Autodesk Fusion 360 part; units mm, degrees
(part 3 of 5)
sketch "LED pad connection profile" plane through (0, 0, -7.475) normal (0, 0, 1) x (1, 0, 0) in component "04 Optical retainer"
  line L0 (38.5, 5.2) -> (41.5, 5.2)
  line L1 (41.5, 5.2) -> (41.5, 11.2)
  line L2 (41.5, 11.2) -> (38.5, 11.2)
  line L3 (38.5, 11.2) -> (38.5, 5.2)
  dimension "d475" = 3
  dimension "d476" = 6
  measures "d475" horizontal distance of L0.start L0.end
  measures "d476" vertical distance of L0.end L1.end
extrude "LED pad connection" add sketch "LED pad connection profile" against normal blind 1.6 separate body makes body 56 in component "04 Optical retainer"
ref_plane "WorkPlane6" through (0, 0, -7.475) normal (0, 0, 1) x (1, 0, 0) in component "04 Optical retainer"
sketch "LED pad connection profile (1)" plane through (0, 0, -7.475) normal (0, 0, 1) x (1, 0, 0) in component "04 Optical retainer"
  line L0 (38.5, 48.8) -> (41.5, 48.8)
  line L1 (41.5, 48.8) -> (41.5, 54.8)
  line L2 (41.5, 54.8) -> (38.5, 54.8)
  line L3 (38.5, 54.8) -> (38.5, 48.8)
  dimension "d481" = 3
  dimension "d482" = 6
  measures "d481" horizontal distance of L0.start L0.end
  measures "d482" vertical distance of L0.end L1.end
extrude "LED pad connection (1)" add sketch "LED pad connection profile (1)" against normal blind 1.6 separate body makes body 57 in component "04 Optical retainer"
ref_plane "WorkPlane7" through (0, 0, -4.35) normal (0, 0, 1) x (1, 0, 0) in component "04 Optical retainer"
sketch "LED hold-down pad profile" plane through (0, 0, -4.35) normal (0, 0, 1) x (1, 0, 0) in component "04 Optical retainer"
  line L0 (38.5, 5.2) -> (41.5, 5.2)
  line L1 (41.5, 5.2) -> (41.5, 10.8)
  line L2 (41.5, 10.8) -> (38.5, 10.8)
  line L3 (38.5, 10.8) -> (38.5, 5.2)
  dimension "d487" = 3
  dimension "d488" = 5.6
  measures "d487" horizontal distance of L0.start L0.end
  measures "d488" vertical distance of L0.end L1.end
extrude "LED hold-down pad" add sketch "LED hold-down pad profile" against normal blind 3.125 separate body makes body 58 in component "04 Optical retainer"
ref_plane "WorkPlane8" through (0, 0, -4.35) normal (0, 0, 1) x (1, 0, 0) in component "04 Optical retainer"
sketch "LED hold-down pad profile (1)" plane through (0, 0, -4.35) normal (0, 0, 1) x (1, 0, 0) in component "04 Optical retainer"
  line L0 (38.5, 49.2) -> (41.5, 49.2)
  line L1 (41.5, 49.2) -> (41.5, 54.8)
  line L2 (41.5, 54.8) -> (38.5, 54.8)
  line L3 (38.5, 54.8) -> (38.5, 49.2)
  dimension "d493" = 3
  dimension "d494" = 5.6
  measures "d493" horizontal distance of L0.start L0.end
  measures "d494" vertical distance of L0.end L1.end
extrude "LED hold-down pad (1)" add sketch "LED hold-down pad profile (1)" against normal blind 3.125 separate body makes body 59 in component "04 Optical retainer"
ref_plane "WorkPlane9" through (0, 0, -7.475) normal (0, 0, 1) x (1, 0, 0) in component "04 Optical retainer"
sketch "LED pad connection profile (2)" plane through (0, 0, -7.475) normal (0, 0, 1) x (1, 0, 0) in component "04 Optical retainer"
  line L0 (78.5, 5.2) -> (81.5, 5.2)
  line L1 (81.5, 5.2) -> (81.5, 11.2)
  line L2 (81.5, 11.2) -> (78.5, 11.2)
  line L3 (78.5, 11.2) -> (78.5, 5.2)
  dimension "d499" = 3
  dimension "d500" = 6
  measures "d499" horizontal distance of L0.start L0.end
  measures "d500" vertical distance of L0.end L1.end
extrude "LED pad connection (2)" add sketch "LED pad connection profile (2)" against normal blind 1.6 separate body makes body 60 in component "04 Optical retainer"
ref_plane "WorkPlane10" through (0, 0, -7.475) normal (0, 0, 1) x (1, 0, 0) in component "04 Optical retainer"
sketch "LED pad connection profile (3)" plane through (0, 0, -7.475) normal (0, 0, 1) x (1, 0, 0) in component "04 Optical retainer"
  line L0 (78.5, 48.8) -> (81.5, 48.8)
  line L1 (81.5, 48.8) -> (81.5, 54.8)
  line L2 (81.5, 54.8) -> (78.5, 54.8)
  line L3 (78.5, 54.8) -> (78.5, 48.8)
  dimension "d505" = 3
  dimension "d506" = 6
  measures "d505" horizontal distance of L0.start L0.end
  measures "d506" vertical distance of L0.end L1.end
extrude "LED pad connection (3)" add sketch "LED pad connection profile (3)" against normal blind 1.6 separate body makes body 61 in component "04 Optical retainer"
ref_plane "WorkPlane11" through (0, 0, -4.35) normal (0, 0, 1) x (1, 0, 0) in component "04 Optical retainer"
sketch "LED hold-down pad profile (2)" plane through (0, 0, -4.35) normal (0, 0, 1) x (1, 0, 0) in component "04 Optical retainer"
  line L0 (78.5, 5.2) -> (81.5, 5.2)
  line L1 (81.5, 5.2) -> (81.5, 10.8)
  line L2 (81.5, 10.8) -> (78.5, 10.8)
  line L3 (78.5, 10.8) -> (78.5, 5.2)
  dimension "d511" = 3
  dimension "d512" = 5.6
  measures "d511" horizontal distance of L0.start L0.end
  measures "d512" vertical distance of L0.end L1.end
extrude "LED hold-down pad (2)" add sketch "LED hold-down pad profile (2)" against normal blind 3.125 separate body makes body 62 in component "04 Optical retainer"
ref_plane "WorkPlane12" through (0, 0, -4.35) normal (0, 0, 1) x (1, 0, 0) in component "04 Optical retainer"
sketch "LED hold-down pad profile (3)" plane through (0, 0, -4.35) normal (0, 0, 1) x (1, 0, 0) in component "04 Optical retainer"
  line L0 (78.5, 49.2) -> (81.5, 49.2)
  line L1 (81.5, 49.2) -> (81.5, 54.8)
  line L2 (81.5, 54.8) -> (78.5, 54.8)
  line L3 (78.5, 54.8) -> (78.5, 49.2)
  dimension "d517" = 3
  dimension "d518" = 5.6
  measures "d517" horizontal distance of L0.start L0.end
  measures "d518" vertical distance of L0.end L1.end
extrude "LED hold-down pad (3)" add sketch "LED hold-down pad profile (3)" against normal blind 3.125 separate body makes body 63 in component "04 Optical retainer"
combine "Union manufactured solid''" operation add target body 53 tool bodies 54 55 56 57 58 59 60 61 62 63 in component "04 Optical retainer"
ref_plane "WorkPlane13" through (0, 0, -7.455) normal (0, 0, 1) x (1, 0, 0) in component "04 Optical retainer"
sketch "Optical M3 clearance profile" plane through (0, 0, -7.455) normal (0, 0, 1) x (1, 0, 0) in component "04 Optical retainer"
  circle A0 centre (60, 6) radius 1.7
  dimension "d523" = 3.4
  measures "d523" diameter of A0
extrude "Optical M3 clearance" cut sketch "Optical M3 clearance profile" against normal blind 1.64 bodies 53 in component "04 Optical retainer"
ref_plane "WorkPlane14" through (0, 0, -7.455) normal (0, 0, 1) x (1, 0, 0) in component "04 Optical retainer"
sketch "Optical M3 clearance profile (1)" plane through (0, 0, -7.455) normal (0, 0, 1) x (1, 0, 0) in component "04 Optical retainer"
  circle A0 centre (60, 54) radius 1.7
  dimension "d528" = 3.4
  measures "d528" diameter of A0
extrude "Optical M3 clearance (1)" cut sketch "Optical M3 clearance profile (1)" against normal blind 1.64 bodies 53 in component "04 Optical retainer"
ref_plane "WorkPlane1" through (0, 0, -4.775) normal (0, 0, 1) x (1, 0, 0) in component "81 Laminate front spacer"
sketch "Laminate front spacer" plane through (0, 0, -4.775) normal (0, 0, 1) x (1, 0, 0) in component "81 Laminate front spacer"
  line L0 (8, 11) -> (112, 11)
  line L1 (112, 11) -> (112, 49)
  line L2 (112, 49) -> (11, 49)
  line L3 (11, 49) -> (8, 46)
  line L4 (8, 46) -> (8, 11)
extrude "Laminate front spacer (1)" add sketch "Laminate front spacer" against normal blind 0.5 separate body makes body 64 in component "81 Laminate front spacer"
ref_plane "WorkPlane2" through (0, 0, -4.765) normal (0, 0, 1) x (1, 0, 0) in component "81 Laminate front spacer"
sketch "Hidden border opening profile" plane through (0, 0, -4.765) normal (0, 0, 1) x (1, 0, 0) in component "81 Laminate front spacer"
  line L0 (9.5, 12.5) -> (110.5, 12.5)
  line L1 (110.5, 12.5) -> (110.5, 47.5)
  line L2 (110.5, 47.5) -> (9.5, 47.5)
  line L3 (9.5, 47.5) -> (9.5, 12.5)
  dimension "d537" = 101
  dimension "d538" = 35
  measures "d537" horizontal distance of L0.start L0.end
  measures "d538" vertical distance of L0.end L1.end
extrude "Hidden border opening" cut sketch "Hidden border opening profile" against normal blind 0.52 bodies 64 in component "81 Laminate front spacer"
ref_plane "WorkPlane1" through (0, 0, -6.875) normal (0, 0, 1) x (1, 0, 0) in component "82 Laminate rear shim"
sketch "Laminate rear shim" plane through (0, 0, -6.875) normal (0, 0, 1) x (1, 0, 0) in component "82 Laminate rear shim"
  line L0 (8, 11) -> (112, 11)
  line L1 (112, 11) -> (112, 49)
  line L2 (112, 49) -> (11, 49)
  line L3 (11, 49) -> (8, 46)
  line L4 (8, 46) -> (8, 11)
extrude "Laminate rear shim (1)" add sketch "Laminate rear shim" against normal blind 0.4 separate body makes body 65 in component "82 Laminate rear shim"
ref_plane "WorkPlane2" through (0, 0, -6.865) normal (0, 0, 1) x (1, 0, 0) in component "82 Laminate rear shim"
sketch "Hidden border opening profile (2)" plane through (0, 0, -6.865) normal (0, 0, 1) x (1, 0, 0) in component "82 Laminate rear shim"
  line L0 (9.5, 12.5) -> (110.5, 12.5)
  line L1 (110.5, 12.5) -> (110.5, 47.5)
  line L2 (110.5, 47.5) -> (9.5, 47.5)
  line L3 (9.5, 47.5) -> (9.5, 12.5)
  dimension "d547" = 101
  dimension "d548" = 35
  measures "d547" horizontal distance of L0.start L0.end
  measures "d548" vertical distance of L0.end L1.end
extrude "Hidden border opening'" cut sketch "Hidden border opening profile (2)" against normal blind 0.42 bodies 65 in component "82 Laminate rear shim"
ref_plane "WorkPlane1" through (0, 0, -9.5) normal (0, 0, 1) x (1, 0, 0) in component "05 Rear electronics housing"
sketch "Rear housing envelope profile" plane through (0, 0, -9.5) normal (0, 0, 1) x (1, 0, 0) in component "05 Rear electronics housing"
  line L0 (3, 0) -> (117, 0)
  line L1 (120, 3) -> (120, 57)
  line L2 (117, 60) -> (3, 60)
  line L3 (0, 57) -> (0, 3)
  arc A0 (117, 0) -> (120, 3) centre (117, 3) ccw
  arc A1 (120, 57) -> (117, 60) centre (117, 57) ccw
  arc A2 (3, 60) -> (0, 57) centre (3, 57) ccw
  arc A3 (0, 3) -> (3, 0) centre (3, 3) ccw
extrude "Rear housing envelope" add sketch "Rear housing envelope profile" against normal blind 24.5 separate body makes body 66 in component "05 Rear electronics housing"
ref_plane "WorkPlane2" through (0, 0, -9.48) normal (0, 0, 1) x (1, 0, 0) in component "05 Rear electronics housing"
sketch "Front open electronics cavity profile" plane through (0, 0, -9.48) normal (0, 0, 1) x (1, 0, 0) in component "05 Rear electronics housing"
  line L0 (2.4, 2.4) -> (117.6, 2.4)
  line L1 (117.6, 2.4) -> (117.6, 57.6)
  line L2 (117.6, 57.6) -> (2.4, 57.6)
  line L3 (2.4, 57.6) -> (2.4, 2.4)
  dimension "d557" = 115.2
  dimension "d558" = 55.2
  measures "d557" horizontal distance of L0.start L0.end
  measures "d558" vertical distance of L0.end L1.end
extrude "Front open electronics cavity" cut sketch "Front open electronics cavity profile" against normal blind 22.12 bodies 66 in component "05 Rear electronics housing"
ref_plane "WorkPlane3" through (0, 0, -9.5) normal (0, 0, 1) x (1, 0, 0) in component "05 Rear electronics housing"
sketch "Closure boss profile" plane through (0, 0, -9.5) normal (0, 0, 1) x (1, 0, 0) in component "05 Rear electronics housing"
  line L0 (1.8, 1.8) -> (10.2, 1.8)
  line L1 (10.2, 1.8) -> (10.2, 10.2)
  line L2 (10.2, 10.2) -> (1.8, 10.2)
  line L3 (1.8, 10.2) -> (1.8, 1.8)
  dimension "d563" = 8.4
  dimension "d564" = 8.4
  measures "d563" horizontal distance of L0.start L0.end
  measures "d564" vertical distance of L0.end L1.end
extrude "Closure boss" add sketch "Closure boss profile" against normal blind 22.2 separate body makes body 67 in component "05 Rear electronics housing"
combine "Union manufactured solid'''" operation add target body 66 tool bodies 67 in component "05 Rear electronics housing"
ref_plane "WorkPlane4" through (0, 0, -24.8) normal (0, 0, 1) x (1, 0, 0) in component "05 Rear electronics housing"
sketch "Closure boss hex pocket" plane through (0, 0, -24.8) normal (0, 0, 1) x (1, 0, 0) in component "05 Rear electronics housing"
  line L0 (9.3486, 6) -> (7.6743, 8.9)
  line L1 (7.6743, 8.9) -> (4.3257, 8.9)
  line L2 (4.3257, 8.9) -> (2.6514, 6)
  line L3 (2.6514, 6) -> (4.3257, 3.1)
  line L4 (4.3257, 3.1) -> (7.6743, 3.1)
  line L5 (7.6743, 3.1) -> (9.3486, 6)
extrude "Closure boss hex pocket (1)" cut sketch "Closure boss hex pocket" against normal blind 2.6 bodies 66 in component "05 Rear electronics housing"
ref_plane "WorkPlane5" through (0, 0, -24.8) normal (0, 0, 1) x (1, 0, 0) in component "05 Rear electronics housing"
sketch "Closure boss side nut entry profile" plane through (0, 0, -24.8) normal (0, 0, 1) x (1, 0, 0) in component "05 Rear electronics housing"
  line L0 (6, 3.1) -> (10.5, 3.1)
  line L1 (10.5, 3.1) -> (10.5, 8.9)
  line L2 (10.5, 8.9) -> (6, 8.9)
  line L3 (6, 8.9) -> (6, 3.1)
  dimension "d573" = 4.5
  dimension "d574" = 5.8
  measures "d573" horizontal distance of L0.start L0.end
  measures "d574" vertical distance of L0.end L1.end
extrude "Closure boss side nut entry" cut sketch "Closure boss side nut entry profile" against normal blind 2.6 bodies 66 in component "05 Rear electronics housing"
ref_plane "WorkPlane6" through (0, 0, -9.48) normal (0, 0, 1) x (1, 0, 0) in component "05 Rear electronics housing"
sketch "Closure boss blind bore profile" plane through (0, 0, -9.48) normal (0, 0, 1) x (1, 0, 0) in component "05 Rear electronics housing"
  circle A0 centre (6, 6) radius 1.7
  dimension "d579" = 3.4
  measures "d579" diameter of A0
extrude "Closure boss blind bore" cut sketch "Closure boss blind bore profile" against normal blind 19.72 bodies 66 in component "05 Rear electronics housing"
ref_plane "WorkPlane7" through (0, 0, -9.5) normal (0, 0, 1) x (1, 0, 0) in component "05 Rear electronics housing"
sketch "Closure boss profile (1)" plane through (0, 0, -9.5) normal (0, 0, 1) x (1, 0, 0) in component "05 Rear electronics housing"
  line L0 (109.8, 1.8) -> (118.2, 1.8)
  line L1 (118.2, 1.8) -> (118.2, 10.2)
  line L2 (118.2, 10.2) -> (109.8, 10.2)
  line L3 (109.8, 10.2) -> (109.8, 1.8)
  dimension "d584" = 8.4
  dimension "d585" = 8.4
  measures "d584" horizontal distance of L0.start L0.end
  measures "d585" vertical distance of L0.end L1.end
extrude "Closure boss (1)" add sketch "Closure boss profile (1)" against normal blind 22.2 separate body makes body 68 in component "05 Rear electronics housing"
combine "Union manufactured solid (1)''" operation add target body 66 tool bodies 68 in component "05 Rear electronics housing"
ref_plane "WorkPlane8" through (0, 0, -24.8) normal (0, 0, 1) x (1, 0, 0) in component "05 Rear electronics housing"
sketch "Closure boss hex pocket (1)" plane through (0, 0, -24.8) normal (0, 0, 1) x (1, 0, 0) in component "05 Rear electronics housing"
  line L0 (117.3486, 6) -> (115.6743, 8.9)
  line L1 (115.6743, 8.9) -> (112.3257, 8.9)
  line L2 (112.3257, 8.9) -> (110.6514, 6)
  line L3 (110.6514, 6) -> (112.3257, 3.1)
  line L4 (112.3257, 3.1) -> (115.6743, 3.1)
  line L5 (115.6743, 3.1) -> (117.3486, 6)
extrude "Closure boss hex pocket (2)" cut sketch "Closure boss hex pocket (1)" against normal blind 2.6 bodies 66 in component "05 Rear electronics housing"
ref_plane "WorkPlane9" through (0, 0, -24.8) normal (0, 0, 1) x (1, 0, 0) in component "05 Rear electronics housing"
sketch "Closure boss side nut entry profile (1)" plane through (0, 0, -24.8) normal (0, 0, 1) x (1, 0, 0) in component "05 Rear electronics housing"
  line L0 (109.5, 3.1) -> (114, 3.1)
  line L1 (114, 3.1) -> (114, 8.9)
  line L2 (114, 8.9) -> (109.5, 8.9)
  line L3 (109.5, 8.9) -> (109.5, 3.1)
  dimension "d594" = 4.5
  dimension "d595" = 5.8
  measures "d594" horizontal distance of L0.start L0.end
  measures "d595" vertical distance of L0.end L1.end
extrude "Closure boss side nut entry (1)" cut sketch "Closure boss side nut entry profile (1)" against normal blind 2.6 bodies 66 in component "05 Rear electronics housing"
ref_plane "WorkPlane10" through (0, 0, -9.48) normal (0, 0, 1) x (1, 0, 0) in component "05 Rear electronics housing"
sketch "Closure boss blind bore profile (1)" plane through (0, 0, -9.48) normal (0, 0, 1) x (1, 0, 0) in component "05 Rear electronics housing"
  circle A0 centre (114, 6) radius 1.7
  dimension "d600" = 3.4
  measures "d600" diameter of A0
extrude "Closure boss blind bore (1)" cut sketch "Closure boss blind bore profile (1)" against normal blind 19.72 bodies 66 in component "05 Rear electronics housing"
ref_plane "WorkPlane11" through (0, 0, -9.5) normal (0, 0, 1) x (1, 0, 0) in component "05 Rear electronics housing"
sketch "Closure boss profile (2)" plane through (0, 0, -9.5) normal (0, 0, 1) x (1, 0, 0) in component "05 Rear electronics housing"
  line L0 (1.8, 49.8) -> (10.2, 49.8)
  line L1 (10.2, 49.8) -> (10.2, 58.2)
  line L2 (10.2, 58.2) -> (1.8, 58.2)
  line L3 (1.8, 58.2) -> (1.8, 49.8)
  dimension "d605" = 8.4
  dimension "d606" = 8.4
  measures "d605" horizontal distance of L0.start L0.end
  measures "d606" vertical distance of L0.end L1.end
extrude "Closure boss (2)" add sketch "Closure boss profile (2)" against normal blind 22.2 separate body makes body 69 in component "05 Rear electronics housing"
combine "Union manufactured solid (2)'" operation add target body 66 tool bodies 69 in component "05 Rear electronics housing"
ref_plane "WorkPlane12" through (0, 0, -24.8) normal (0, 0, 1) x (1, 0, 0) in component "05 Rear electronics housing"
sketch "Closure boss hex pocket (2)" plane through (0, 0, -24.8) normal (0, 0, 1) x (1, 0, 0) in component "05 Rear electronics housing"
  line L0 (9.3486, 54) -> (7.6743, 56.9)
  line L1 (7.6743, 56.9) -> (4.3257, 56.9)
  line L2 (4.3257, 56.9) -> (2.6514, 54)
  line L3 (2.6514, 54) -> (4.3257, 51.1)
  line L4 (4.3257, 51.1) -> (7.6743, 51.1)
  line L5 (7.6743, 51.1) -> (9.3486, 54)
extrude "Closure boss hex pocket (3)" cut sketch "Closure boss hex pocket (2)" against normal blind 2.6 bodies 66 in component "05 Rear electronics housing"
ref_plane "WorkPlane13" through (0, 0, -24.8) normal (0, 0, 1) x (1, 0, 0) in component "05 Rear electronics housing"
sketch "Closure boss side nut entry profile (2)" plane through (0, 0, -24.8) normal (0, 0, 1) x (1, 0, 0) in component "05 Rear electronics housing"
  line L0 (6, 51.1) -> (10.5, 51.1)
  line L1 (10.5, 51.1) -> (10.5, 56.9)
  line L2 (10.5, 56.9) -> (6, 56.9)
  line L3 (6, 56.9) -> (6, 51.1)
  dimension "d615" = 4.5
  dimension "d616" = 5.8
  measures "d615" horizontal distance of L0.start L0.end
  measures "d616" vertical distance of L0.end L1.end
extrude "Closure boss side nut entry (2)" cut sketch "Closure boss side nut entry profile (2)" against normal blind 2.6 bodies 66 in component "05 Rear electronics housing"
ref_plane "WorkPlane14" through (0, 0, -9.48) normal (0, 0, 1) x (1, 0, 0) in component "05 Rear electronics housing"
sketch "Closure boss blind bore profile (2)" plane through (0, 0, -9.48) normal (0, 0, 1) x (1, 0, 0) in component "05 Rear electronics housing"
  circle A0 centre (6, 54) radius 1.7
  dimension "d621" = 3.4
  measures "d621" diameter of A0
extrude "Closure boss blind bore (2)" cut sketch "Closure boss blind bore profile (2)" against normal blind 19.72 bodies 66 in component "05 Rear electronics housing"
ref_plane "WorkPlane15" through (0, 0, -9.5) normal (0, 0, 1) x (1, 0, 0) in component "05 Rear electronics housing"
sketch "Closure boss profile (3)" plane through (0, 0, -9.5) normal (0, 0, 1) x (1, 0, 0) in component "05 Rear electronics housing"
  line L0 (91.8, 49.8) -> (100.2, 49.8)
  line L1 (100.2, 49.8) -> (100.2, 58.2)
  line L2 (100.2, 58.2) -> (91.8, 58.2)
  line L3 (91.8, 58.2) -> (91.8, 49.8)
  dimension "d626" = 8.4
  dimension "d627" = 8.4
  measures "d626" horizontal distance of L0.start L0.end
  measures "d627" vertical distance of L0.end L1.end
extrude "Closure boss (3)" add sketch "Closure boss profile (3)" against normal blind 22.2 separate body makes body 70 in component "05 Rear electronics housing"
combine "Union manufactured solid (3)" operation add target body 66 tool bodies 70 in component "05 Rear electronics housing"
ref_plane "WorkPlane16" through (0, 0, -24.8) normal (0, 0, 1) x (1, 0, 0) in component "05 Rear electronics housing"
sketch "Closure boss hex pocket (3)" plane through (0, 0, -24.8) normal (0, 0, 1) x (1, 0, 0) in component "05 Rear electronics housing"
  line L0 (99.3486, 54) -> (97.6743, 56.9)
  line L1 (97.6743, 56.9) -> (94.3257, 56.9)
  line L2 (94.3257, 56.9) -> (92.6514, 54)
  line L3 (92.6514, 54) -> (94.3257, 51.1)
  line L4 (94.3257, 51.1) -> (97.6743, 51.1)
  line L5 (97.6743, 51.1) -> (99.3486, 54)
extrude "Closure boss hex pocket (4)" cut sketch "Closure boss hex pocket (3)" against normal blind 2.6 bodies 66 in component "05 Rear electronics housing"
ref_plane "WorkPlane17" through (0, 0, -24.8) normal (0, 0, 1) x (1, 0, 0) in component "05 Rear electronics housing"
sketch "Closure boss side nut entry profile (3)" plane through (0, 0, -24.8) normal (0, 0, 1) x (1, 0, 0) in component "05 Rear electronics housing"
  line L0 (91.5, 51.1) -> (96, 51.1)
  line L1 (96, 51.1) -> (96, 56.9)
  line L2 (96, 56.9) -> (91.5, 56.9)
  line L3 (91.5, 56.9) -> (91.5, 51.1)
  dimension "d636" = 4.5
  dimension "d637" = 5.8
  measures "d636" horizontal distance of L0.start L0.end
  measures "d637" vertical distance of L0.end L1.end
extrude "Closure boss side nut entry (3)" cut sketch "Closure boss side nut entry profile (3)" against normal blind 2.6 bodies 66 in component "05 Rear electronics housing"
ref_plane "WorkPlane18" through (0, 0, -9.48) normal (0, 0, 1) x (1, 0, 0) in component "05 Rear electronics housing"
sketch "Closure boss blind bore profile (3)" plane through (0, 0, -9.48) normal (0, 0, 1) x (1, 0, 0) in component "05 Rear electronics housing"
  circle A0 centre (96, 54) radius 1.7
  dimension "d642" = 3.4
  measures "d642" diameter of A0
extrude "Closure boss blind bore (3)" cut sketch "Closure boss blind bore profile (3)" against normal blind 19.72 bodies 66 in component "05 Rear electronics housing"
ref_plane "WorkPlane19" through (0, 0, -27.1) normal (0, 0, 1) x (1, 0, 0) in component "05 Rear electronics housing"
sketch "Battery fence profile" plane through (0, 0, -27.1) normal (0, 0, 1) x (1, 0, 0) in component "05 Rear electronics housing"
  line L0 (32.4, 8.4) -> (89.6, 8.4)
  line L1 (89.6, 8.4) -> (89.6, 10)
  line L2 (89.6, 10) -> (32.4, 10)
  line L3 (32.4, 10) -> (32.4, 8.4)
  dimension "d647" = 57.2
  dimension "d648" = 1.6
  measures "d647" horizontal distance of L0.start L0.end
  measures "d648" vertical distance of L0.end L1.end
extrude "Battery fence" add sketch "Battery fence profile" against normal blind 4.6 separate body makes body 71 in component "05 Rear electronics housing"
ref_plane "WorkPlane20" through (0, 0, -27.1) normal (0, 0, 1) x (1, 0, 0) in component "05 Rear electronics housing"
sketch "Battery fence profile (1)" plane through (0, 0, -27.1) normal (0, 0, 1) x (1, 0, 0) in component "05 Rear electronics housing"
  line L0 (32.4, 10) -> (34, 10)
  line L1 (34, 10) -> (34, 33)
  line L2 (34, 33) -> (32.4, 33)
  line L3 (32.4, 33) -> (32.4, 10)
  dimension "d653" = 1.6
  dimension "d654" = 23
  measures "d653" horizontal distance of L0.start L0.end
  measures "d654" vertical distance of L0.end L1.end
extrude "Battery fence (1)" add sketch "Battery fence profile (1)" against normal blind 4.6 separate body makes body 72 in component "05 Rear electronics housing"
ref_plane "WorkPlane21" through (0, 0, -27.1) normal (0, 0, 1) x (1, 0, 0) in component "05 Rear electronics housing"
sketch "Battery fence profile (2)" plane through (0, 0, -27.1) normal (0, 0, 1) x (1, 0, 0) in component "05 Rear electronics housing"
  line L0 (88, 10) -> (89.6, 10)
  line L1 (89.6, 10) -> (89.6, 27)
  line L2 (89.6, 27) -> (88, 27)
  line L3 (88, 27) -> (88, 10)
  dimension "d659" = 1.6
  dimension "d660" = 17
  measures "d659" horizontal distance of L0.start L0.end
  measures "d660" vertical distance of L0.end L1.end
extrude "Battery fence (2)" add sketch "Battery fence profile (2)" against normal blind 4.6 separate body makes body 73 in component "05 Rear electronics housing"
ref_plane "WorkPlane22" through (0, 0, -27.1) normal (0, 0, 1) x (1, 0, 0) in component "05 Rear electronics housing"
sketch "Battery fence profile (3)" plane through (0, 0, -27.1) normal (0, 0, 1) x (1, 0, 0) in component "05 Rear electronics housing"
  line L0 (34, 33) -> (74, 33)
  line L1 (74, 33) -> (74, 34.6)
  line L2 (74, 34.6) -> (34, 34.6)
  line L3 (34, 34.6) -> (34, 33)
  dimension "d665" = 40
  dimension "d666" = 1.6
  measures "d665" horizontal distance of L0.start L0.end
  measures "d666" vertical distance of L0.end L1.end
extrude "Battery fence (3)" add sketch "Battery fence profile (3)" against normal blind 4.6 separate body makes body 74 in component "05 Rear electronics housing"
ref_plane "WorkPlane23" through (0, 0, -31.3) normal (0, 0, 1) x (1, 0, 0) in component "05 Rear electronics housing"
sketch "Battery bed profile" plane through (0, 0, -31.3) normal (0, 0, 1) x (1, 0, 0) in component "05 Rear electronics housing"
  line L0 (34, 10) -> (88, 10)
  line L1 (88, 10) -> (88, 33)
  line L2 (88, 33) -> (34, 33)
  line L3 (34, 33) -> (34, 10)
  dimension "d671" = 54
  dimension "d672" = 23
  measures "d671" horizontal distance of L0.start L0.end
  measures "d672" vertical distance of L0.end L1.end
extrude "Battery bed" add sketch "Battery bed profile" against normal blind 0.4 separate body makes body 75 in component "05 Rear electronics housing"
ref_plane "WorkPlane24" through (0, 0, -25.2) normal (0, 0, 1) x (1, 0, 0) in component "05 Rear electronics housing"
sketch "Raised strap lug profile" plane through (0, 0, -25.2) normal (0, 0, 1) x (1, 0, 0) in component "05 Rear electronics housing"
  line L0 (28.4, 18) -> (32.4, 18)
  line L1 (32.4, 18) -> (32.4, 25)
  line L2 (32.4, 25) -> (28.4, 25)
  line L3 (28.4, 25) -> (28.4, 18)
  dimension "d677" = 4
  dimension "d678" = 7
  measures "d677" horizontal distance of L0.start L0.end
  measures "d678" vertical distance of L0.end L1.end
extrude "Raised strap lug" add sketch "Raised strap lug profile" against normal blind 6.5 separate body makes body 76 in component "05 Rear electronics housing"
ref_plane "WorkPlane25" through (0, 0, -25.2) normal (0, 0, 1) x (1, 0, 0) in component "05 Rear electronics housing"
sketch "Raised strap lug profile (1)" plane through (0, 0, -25.2) normal (0, 0, 1) x (1, 0, 0) in component "05 Rear electronics housing"
  line L0 (90, 18) -> (94, 18)
  line L1 (94, 18) -> (94, 25)
  line L2 (94, 25) -> (90, 25)
  line L3 (90, 25) -> (90, 18)
  dimension "d683" = 4
  dimension "d684" = 7
  measures "d683" horizontal distance of L0.start L0.end
  measures "d684" vertical distance of L0.end L1.end
extrude "Raised strap lug (1)" add sketch "Raised strap lug profile (1)" against normal blind 6.5 separate body makes body 77 in component "05 Rear electronics housing"
combine "Union manufactured solid (4)" operation add target body 66 tool bodies 71 72 73 74 75 76 77 in component "05 Rear electronics housing"
ref_plane "WorkPlane26" through (28.3, 0, 0) normal (1, 0, 0) x (0, 1, 0) in component "05 Rear electronics housing"
sketch "Strap slot with tent roof" plane through (28.3, 0, 0) normal (1, 0, 0) x (0, 0, -1) in component "05 Rear electronics housing"
  line L0 (30.4, 20) -> (30.4, 23)
  line L1 (30.4, 23) -> (28.8, 23)
  line L2 (28.8, 23) -> (27.3, 21.5)
  line L3 (27.3, 21.5) -> (28.8, 20)
  line L4 (28.8, 20) -> (30.4, 20)
extrude "Strap slot with tent roof (1)" cut sketch "Strap slot with tent roof" along normal blind 4.2 bodies 66 in component "05 Rear electronics housing"
ref_plane "WorkPlane27" through (89.9, 0, 0) normal (1, 0, 0) x (0, 1, 0) in component "05 Rear electronics housing"
sketch "Strap slot with tent roof (1)" plane through (89.9, 0, 0) normal (1, 0, 0) x (0, 0, -1) in component "05 Rear electronics housing"
  line L0 (30.4, 20) -> (30.4, 23)
  line L1 (30.4, 23) -> (28.8, 23)
  line L2 (28.8, 23) -> (27.3, 21.5)
  line L3 (27.3, 21.5) -> (28.8, 20)
  line L4 (28.8, 20) -> (30.4, 20)
extrude "Strap slot with tent roof (2)" cut sketch "Strap slot with tent roof (1)" along normal blind 4.2 bodies 66 in component "05 Rear electronics housing"
ref_plane "WorkPlane28" through (0, 0, -24.2) normal (0, 0, 1) x (1, 0, 0) in component "05 Rear electronics housing"
sketch "Charger PCB seat profile" plane through (0, 0, -24.2) normal (0, 0, 1) x (1, 0, 0) in component "05 Rear electronics housing"
  line L0 (13.1, 34) -> (15.1, 34)
  line L1 (15.1, 34) -> (15.1, 36)
  line L2 (15.1, 36) -> (13.1, 36)
  line L3 (13.1, 36) -> (13.1, 34)
  dimension "d697" = 2
  dimension "d698" = 2
  measures "d697" horizontal distance of L0.start L0.end
  measures "d698" vertical distance of L0.end L1.end
extrude "Charger PCB seat" add sketch "Charger PCB seat profile" against normal blind 7.5 separate body makes body 78 in component "05 Rear electronics housing"
ref_plane "WorkPlane29" through (0, 0, -24.2) normal (0, 0, 1) x (1, 0, 0) in component "05 Rear electronics housing"
sketch "Charger PCB seat profile (1)" plane through (0, 0, -24.2) normal (0, 0, 1) x (1, 0, 0) in component "05 Rear electronics housing"
  line L0 (26.9, 34) -> (28.9, 34)
  line L1 (28.9, 34) -> (28.9, 36)
  line L2 (28.9, 36) -> (26.9, 36)
  line L3 (26.9, 36) -> (26.9, 34)
  dimension "d703" = 2
  dimension "d704" = 2
  measures "d703" horizontal distance of L0.start L0.end
  measures "d704" vertical distance of L0.end L1.end
extrude "Charger PCB seat (1)" add sketch "Charger PCB seat profile (1)" against normal blind 7.5 separate body makes body 79 in component "05 Rear electronics housing"
ref_plane "WorkPlane30" through (0, 0, -24.2) normal (0, 0, 1) x (1, 0, 0) in component "05 Rear electronics housing"
sketch "Charger PCB seat profile (2)" plane through (0, 0, -24.2) normal (0, 0, 1) x (1, 0, 0) in component "05 Rear electronics housing"
  line L0 (13.1, 51) -> (15.1, 51)
  line L1 (15.1, 51) -> (15.1, 53)
  line L2 (15.1, 53) -> (13.1, 53)
  line L3 (13.1, 53) -> (13.1, 51)
  dimension "d709" = 2
  dimension "d710" = 2
  measures "d709" horizontal distance of L0.start L0.end
  measures "d710" vertical distance of L0.end L1.end
extrude "Charger PCB seat (2)" add sketch "Charger PCB seat profile (2)" against normal blind 7.5 separate body makes body 80 in component "05 Rear electronics housing"
ref_plane "WorkPlane31" through (0, 0, -24.2) normal (0, 0, 1) x (1, 0, 0) in component "05 Rear electronics housing"
sketch "Charger PCB seat profile (3)" plane through (0, 0, -24.2) normal (0, 0, 1) x (1, 0, 0) in component "05 Rear electronics housing"
  line L0 (26.9, 51) -> (28.9, 51)
  line L1 (28.9, 51) -> (28.9, 53)
  line L2 (28.9, 53) -> (26.9, 53)
  line L3 (26.9, 53) -> (26.9, 51)
  dimension "d715" = 2
  dimension "d716" = 2
  measures "d715" horizontal distance of L0.start L0.end
  measures "d716" vertical distance of L0.end L1.end
extrude "Charger PCB seat (3)" add sketch "Charger PCB seat profile (3)" against normal blind 7.5 separate body makes body 81 in component "05 Rear electronics housing"
ref_plane "WorkPlane32" through (0, 0, -22) normal (0, 0, 1) x (1, 0, 0) in component "05 Rear electronics housing"
sketch "Charger side fence profile" plane through (0, 0, -22) normal (0, 0, 1) x (1, 0, 0) in component "05 Rear electronics housing"
  line L0 (10.65, 31) -> (12.5, 31)
  line L1 (12.5, 31) -> (12.5, 56)
  line L2 (12.5, 56) -> (10.65, 56)
  line L3 (10.65, 56) -> (10.65, 31)
  dimension "d721" = 1.85
  dimension "d722" = 25
  measures "d721" horizontal distance of L0.start L0.end
  measures "d722" vertical distance of L0.end L1.end
extrude "Charger side fence" add sketch "Charger side fence profile" against normal blind 9.7 separate body makes body 82 in component "05 Rear electronics housing"
ref_plane "WorkPlane33" through (0, 0, -22) normal (0, 0, 1) x (1, 0, 0) in component "05 Rear electronics housing"
sketch "Charger side fence profile (1)" plane through (0, 0, -22) normal (0, 0, 1) x (1, 0, 0) in component "05 Rear electronics housing"
  line L0 (29.5, 31) -> (31.35, 31)
  line L1 (31.35, 31) -> (31.35, 56)
  line L2 (31.35, 56) -> (29.5, 56)
  line L3 (29.5, 56) -> (29.5, 31)
  dimension "d727" = 1.85
  dimension "d728" = 25
  measures "d727" horizontal distance of L0.start L0.end
  measures "d728" vertical distance of L0.end L1.end
extrude "Charger side fence (1)" add sketch "Charger side fence profile (1)" against normal blind 9.7 separate body makes body 83 in component "05 Rear electronics housing"
ref_plane "WorkPlane34" through (0, 0, -22) normal (0, 0, 1) x (1, 0, 0) in component "05 Rear electronics housing"
sketch "Charger insertion stop profile" plane through (0, 0, -22) normal (0, 0, 1) x (1, 0, 0) in component "05 Rear electronics housing"
  line L0 (12.5, 30.4) -> (29.5, 30.4)
  line L1 (29.5, 30.4) -> (29.5, 31.75)
  line L2 (29.5, 31.75) -> (12.5, 31.75)
  line L3 (12.5, 31.75) -> (12.5, 30.4)
  dimension "d733" = 17
  dimension "d734" = 1.35
  measures "d733" horizontal distance of L0.start L0.end
  measures "d734" vertical distance of L0.end L1.end
extrude "Charger insertion stop" add sketch "Charger insertion stop profile" against normal blind 9.7 separate body makes body 84 in component "05 Rear electronics housing"
ref_plane "WorkPlane35" through (0, 0, -22) normal (0, 0, 1) x (1, 0, 0) in component "05 Rear electronics housing"
sketch "Charger extraction stop profile" plane through (0, 0, -22) normal (0, 0, 1) x (1, 0, 0) in component "05 Rear electronics housing"
  line L0 (12.5, 57.25) -> (14.5, 57.25)
  line L1 (14.5, 57.25) -> (14.5, 58.25)
  line L2 (14.5, 58.25) -> (12.5, 58.25)
  line L3 (12.5, 58.25) -> (12.5, 57.25)
  dimension "d739" = 2
  dimension "d740" = 1
  measures "d739" horizontal distance of L0.start L0.end
  measures "d740" vertical distance of L0.end L1.end
extrude "Charger extraction stop" add sketch "Charger extraction stop profile" against normal blind 9.7 separate body makes body 85 in component "05 Rear electronics housing"
ref_plane "WorkPlane36" through (0, 0, -22) normal (0, 0, 1) x (1, 0, 0) in component "05 Rear electronics housing"
sketch "Charger extraction stop profile (1)" plane through (0, 0, -22) normal (0, 0, 1) x (1, 0, 0) in component "05 Rear electronics housing"
  line L0 (28.5, 57.25) -> (30.5, 57.25)
  line L1 (30.5, 57.25) -> (30.5, 58.25)
  line L2 (30.5, 58.25) -> (28.5, 58.25)
  line L3 (28.5, 58.25) -> (28.5, 57.25)
  dimension "d745" = 2
  dimension "d746" = 1
  measures "d745" horizontal distance of L0.start L0.end
  measures "d746" vertical distance of L0.end L1.end
extrude "Charger extraction stop (1)" add sketch "Charger extraction stop profile (1)" against normal blind 9.7 separate body makes body 86 in component "05 Rear electronics housing"
ref_plane "WorkPlane37" through (0, 0, -11.4) normal (0, 0, 1) x (1, 0, 0) in component "05 Rear electronics housing"
sketch "XIAO inner spine profile" plane through (0, 0, -11.4) normal (0, 0, 1) x (1, 0, 0) in component "05 Rear electronics housing"
  line L0 (108.9, 35.2) -> (110.75, 35.2)
  line L1 (110.75, 35.2) -> (110.75, 56.8)
  line L2 (110.75, 56.8) -> (108.9, 56.8)
  line L3 (108.9, 56.8) -> (108.9, 35.2)
  dimension "d751" = 1.85
  dimension "d752" = 21.6
  measures "d751" horizontal distance of L0.start L0.end
  measures "d752" vertical distance of L0.end L1.end
extrude "XIAO inner spine" add sketch "XIAO inner spine profile" against normal blind 20.3 separate body makes body 87 in component "05 Rear electronics housing"
ref_plane "WorkPlane38" through (0, 0, -27.65) normal (0, 0, 1) x (1, 0, 0) in component "05 Rear electronics housing"
sketch "XIAO rear outer cheek profile" plane through (0, 0, -27.65) normal (0, 0, 1) x (1, 0, 0) in component "05 Rear electronics housing"
  line L0 (112.25, 35.2) -> (113.75, 35.2)
  line L1 (113.75, 35.2) -> (113.75, 56.8)
  line L2 (113.75, 56.8) -> (112.25, 56.8)
  line L3 (112.25, 56.8) -> (112.25, 35.2)
  dimension "d757" = 1.5
  dimension "d758" = 21.6
  measures "d757" horizontal distance of L0.start L0.end
  measures "d758" vertical distance of L0.end L1.end
extrude "XIAO rear outer cheek" add sketch "XIAO rear outer cheek profile" against normal blind 4.05 separate body makes body 88 in component "05 Rear electronics housing"
ref_plane "WorkPlane39" through (0, 0, -29.6) normal (0, 0, 1) x (1, 0, 0) in component "05 Rear electronics housing"
sketch "XIAO rear depth stop profile" plane through (0, 0, -29.6) normal (0, 0, 1) x (1, 0, 0) in component "05 Rear electronics housing"
  line L0 (110.7, 35.2) -> (113.75, 35.2)
  line L1 (113.75, 35.2) -> (113.75, 56.8)
  line L2 (113.75, 56.8) -> (110.7, 56.8)
  line L3 (110.7, 56.8) -> (110.7, 35.2)
  dimension "d763" = 3.05
  dimension "d764" = 21.6
  measures "d763" horizontal distance of L0.start L0.end
  measures "d764" vertical distance of L0.end L1.end
extrude "XIAO rear depth stop" add sketch "XIAO rear depth stop profile" against normal blind 2.1 separate body makes body 89 in component "05 Rear electronics housing"
ref_plane "WorkPlane40" through (0, 0, -11.4) normal (0, 0, 1) x (1, 0, 0) in component "05 Rear electronics housing"
sketch "XIAO lower axial stop profile" plane through (0, 0, -11.4) normal (0, 0, 1) x (1, 0, 0) in component "05 Rear electronics housing"
  line L0 (110.75, 34) -> (112.25, 34)
  line L1 (112.25, 34) -> (112.25, 35.25)
  line L2 (112.25, 35.25) -> (110.75, 35.25)
  line L3 (110.75, 35.25) -> (110.75, 34)
  dimension "d769" = 1.5
  dimension "d770" = 1.25
  measures "d769" horizontal distance of L0.start L0.end
  measures "d770" vertical distance of L0.end L1.end
extrude "XIAO lower axial stop" add sketch "XIAO lower axial stop profile" against normal blind 20.3 separate body makes body 90 in component "05 Rear electronics housing"
ref_plane "WorkPlane41" through (0, 0, -11.4) normal (0, 0, 1) x (1, 0, 0) in component "05 Rear electronics housing"
sketch "XIAO upper axial stop profile" plane through (0, 0, -11.4) normal (0, 0, 1) x (1, 0, 0) in component "05 Rear electronics housing"
  line L0 (110.75, 56.75) -> (111.75, 56.75)
  line L1 (111.75, 56.75) -> (111.75, 57.9)
  line L2 (111.75, 57.9) -> (110.75, 57.9)
  line L3 (110.75, 57.9) -> (110.75, 56.75)
  dimension "d775" = 1
  dimension "d776" = 1.15
  measures "d775" horizontal distance of L0.start L0.end
  measures "d776" vertical distance of L0.end L1.end
extrude "XIAO upper axial stop" add sketch "XIAO upper axial stop profile" against normal blind 20.3 separate body makes body 91 in component "05 Rear electronics housing"
ref_plane "WorkPlane42" through (0, 0, -23.1) normal (0, 0, 1) x (1, 0, 0) in component "05 Rear electronics housing"
sketch "DPDT rear seat profile" plane through (0, 0, -23.1) normal (0, 0, 1) x (1, 0, 0) in component "05 Rear electronics housing"
  line L0 (55.45, 49.25) -> (64.55, 49.25)
  line L1 (64.55, 49.25) -> (64.55, 52.45)
  line L2 (64.55, 52.45) -> (55.45, 52.45)
  line L3 (55.45, 52.45) -> (55.45, 49.25)
  dimension "d781" = 9.1
  dimension "d782" = 3.2
  measures "d781" horizontal distance of L0.start L0.end
  measures "d782" vertical distance of L0.end L1.end
extrude "DPDT rear seat" add sketch "DPDT rear seat profile" against normal blind 8.6 separate body makes body 92 in component "05 Rear electronics housing"
ref_plane "WorkPlane43" through (0, 0, -19.8) normal (0, 0, 1) x (1, 0, 0) in component "05 Rear electronics housing"
sketch "DPDT side cheek profile" plane through (0, 0, -19.8) normal (0, 0, 1) x (1, 0, 0) in component "05 Rear electronics housing"
  line L0 (54.2, 48) -> (55.45, 48)
  line L1 (55.45, 48) -> (55.45, 53.2)
  line L2 (55.45, 53.2) -> (54.2, 53.2)
  line L3 (54.2, 53.2) -> (54.2, 48)
  dimension "d787" = 1.25
  dimension "d788" = 5.2
  measures "d787" horizontal distance of L0.start L0.end
  measures "d788" vertical distance of L0.end L1.end
extrude "DPDT side cheek" add sketch "DPDT side cheek profile" against normal blind 11.9 separate body makes body 93 in component "05 Rear electronics housing"
ref_plane "WorkPlane44" through (0, 0, -19.8) normal (0, 0, 1) x (1, 0, 0) in component "05 Rear electronics housing"
sketch "DPDT side cheek profile (1)" plane through (0, 0, -19.8) normal (0, 0, 1) x (1, 0, 0) in component "05 Rear electronics housing"
  line L0 (64.55, 48) -> (65.8, 48)
  line L1 (65.8, 48) -> (65.8, 53.2)
  line L2 (65.8, 53.2) -> (64.55, 53.2)
  line L3 (64.55, 53.2) -> (64.55, 48)
  dimension "d793" = 1.25
  dimension "d794" = 5.2
  measures "d793" horizontal distance of L0.start L0.end
  measures "d794" vertical distance of L0.end L1.end
extrude "DPDT side cheek (1)" add sketch "DPDT side cheek profile (1)" against normal blind 11.9 separate body makes body 94 in component "05 Rear electronics housing"
ref_plane "WorkPlane45" through (0, 0, -19.8) normal (0, 0, 1) x (1, 0, 0) in component "05 Rear electronics housing"
sketch "DPDT axial stop profile" plane through (0, 0, -19.8) normal (0, 0, 1) x (1, 0, 0) in component "05 Rear electronics housing"
  line L0 (54.2, 48) -> (56.1, 48)
  line L1 (56.1, 48) -> (56.1, 49.25)
  line L2 (56.1, 49.25) -> (54.2, 49.25)
  line L3 (54.2, 49.25) -> (54.2, 48)
  dimension "d799" = 1.9
  dimension "d800" = 1.25
  measures "d799" horizontal distance of L0.start L0.end
  measures "d800" vertical distance of L0.end L1.end
extrude "DPDT axial stop" add sketch "DPDT axial stop profile" against normal blind 11.9 separate body makes body 95 in component "05 Rear electronics housing"
ref_plane "WorkPlane46" through (0, 0, -19.8) normal (0, 0, 1) x (1, 0, 0) in component "05 Rear electronics housing"
sketch "DPDT axial stop profile (1)" plane through (0, 0, -19.8) normal (0, 0, 1) x (1, 0, 0) in component "05 Rear electronics housing"
  line L0 (54.2, 52.45) -> (56.1, 52.45)
  line L1 (56.1, 52.45) -> (56.1, 53.2)
  line L2 (56.1, 53.2) -> (54.2, 53.2)
  line L3 (54.2, 53.2) -> (54.2, 52.45)
  dimension "d805" = 1.9
  dimension "d806" = 0.75
  measures "d805" horizontal distance of L0.start L0.end
  measures "d806" vertical distance of L0.end L1.end
extrude "DPDT axial stop (1)" add sketch "DPDT axial stop profile (1)" against normal blind 11.9 separate body makes body 96 in component "05 Rear electronics housing"
ref_plane "WorkPlane47" through (0, 0, -19.8) normal (0, 0, 1) x (1, 0, 0) in component "05 Rear electronics housing"
sketch "DPDT axial stop profile (2)" plane through (0, 0, -19.8) normal (0, 0, 1) x (1, 0, 0) in component "05 Rear electronics housing"
  line L0 (63.9, 48) -> (65.8, 48)
  line L1 (65.8, 48) -> (65.8, 49.25)
  line L2 (65.8, 49.25) -> (63.9, 49.25)
  line L3 (63.9, 49.25) -> (63.9, 48)
  dimension "d811" = 1.9
  dimension "d812" = 1.25
  measures "d811" horizontal distance of L0.start L0.end
  measures "d812" vertical distance of L0.end L1.end
extrude "DPDT axial stop (2)" add sketch "DPDT axial stop profile (2)" against normal blind 11.9 separate body makes body 97 in component "05 Rear electronics housing"
ref_plane "WorkPlane48" through (0, 0, -19.8) normal (0, 0, 1) x (1, 0, 0) in component "05 Rear electronics housing"
sketch "DPDT axial stop profile (3)" plane through (0, 0, -19.8) normal (0, 0, 1) x (1, 0, 0) in component "05 Rear electronics housing"
  line L0 (63.9, 52.45) -> (65.8, 52.45)
  line L1 (65.8, 52.45) -> (65.8, 53.2)
  line L2 (65.8, 53.2) -> (63.9, 53.2)
  line L3 (63.9, 53.2) -> (63.9, 52.45)
  dimension "d817" = 1.9
  dimension "d818" = 0.75
  measures "d817" horizontal distance of L0.start L0.end
  measures "d818" vertical distance of L0.end L1.end
extrude "DPDT axial stop (3)" add sketch "DPDT axial stop profile (3)" against normal blind 11.9 separate body makes body 98 in component "05 Rear electronics housing"
combine "Union manufactured solid (5)" operation add target body 66 tool bodies 78 79 80 81 82 83 84 85 86 87 88 89 90 91 92 93 94 95 96 97 98 in component "05 Rear electronics housing"
ref_plane "WorkPlane49" through (0, 0, -11.4) normal (0, 0, 1) x (1, 0, 0) in component "05 Rear electronics housing"
sketch "Yoke mounting boss profile" plane through (0, 0, -11.4) normal (0, 0, 1) x (1, 0, 0) in component "05 Rear electronics housing"
  line L0 (30.8, 33.8) -> (39.2, 33.8)
  line L1 (39.2, 33.8) -> (39.2, 42.2)
  line L2 (39.2, 42.2) -> (30.8, 42.2)
  line L3 (30.8, 42.2) -> (30.8, 33.8)
  dimension "d823" = 8.4
  dimension "d824" = 8.4
  measures "d823" horizontal distance of L0.start L0.end
  measures "d824" vertical distance of L0.end L1.end
extrude "Yoke mounting boss" add sketch "Yoke mounting boss profile" against normal blind 20.3 separate body makes body 99 in component "05 Rear electronics housing"
combine "Union manufactured solid (6)" operation add target body 66 tool bodies 99 in component "05 Rear electronics housing"
ref_plane "WorkPlane50" through (0, 0, -13.8) normal (0, 0, 1) x (1, 0, 0) in component "05 Rear electronics housing"
sketch "Yoke mounting boss hex pocket" plane through (0, 0, -13.8) normal (0, 0, 1) x (1, 0, 0) in component "05 Rear electronics housing"
  line L0 (38.3486, 38) -> (36.6743, 40.9)
  line L1 (36.6743, 40.9) -> (33.3257, 40.9)
  line L2 (33.3257, 40.9) -> (31.6514, 38)
  line L3 (31.6514, 38) -> (33.3257, 35.1)
  line L4 (33.3257, 35.1) -> (36.6743, 35.1)
  line L5 (36.6743, 35.1) -> (38.3486, 38)
extrude "Yoke mounting boss hex pocket (1)" cut sketch "Yoke mounting boss hex pocket" against normal blind 2.6 bodies 66 in component "05 Rear electronics housing"
ref_plane "WorkPlane51" through (0, 0, -13.8) normal (0, 0, 1) x (1, 0, 0) in component "05 Rear electronics housing"
sketch "Yoke mounting boss side nut entry profile" plane through (0, 0, -13.8) normal (0, 0, 1) x (1, 0, 0) in component "05 Rear electronics housing"
  line L0 (30.5, 35.1) -> (35, 35.1)
  line L1 (35, 35.1) -> (35, 40.9)
  line L2 (35, 40.9) -> (30.5, 40.9)
  line L3 (30.5, 40.9) -> (30.5, 35.1)
  dimension "d833" = 4.5
  dimension "d834" = 5.8
  measures "d833" horizontal distance of L0.start L0.end
  measures "d834" vertical distance of L0.end L1.end
extrude "Yoke mounting boss side nut entry" cut sketch "Yoke mounting boss side nut entry profile" against normal blind 2.6 bodies 66 in component "05 Rear electronics housing"
ref_plane "WorkPlane52" through (0, 0, -11.38) normal (0, 0, 1) x (1, 0, 0) in component "05 Rear electronics housing"
sketch "Yoke mounting boss blind bore profile" plane through (0, 0, -11.38) normal (0, 0, 1) x (1, 0, 0) in component "05 Rear electronics housing"
  circle A0 centre (35, 38) radius 1.7
  dimension "d839" = 3.4
  measures "d839" diameter of A0
extrude "Yoke mounting boss blind bore" cut sketch "Yoke mounting boss blind bore profile" against normal blind 6.82 bodies 66 in component "05 Rear electronics housing"
ref_plane "WorkPlane53" through (0, 0, -11.4) normal (0, 0, 1) x (1, 0, 0) in component "05 Rear electronics housing"
sketch "Yoke mounting boss profile (1)" plane through (0, 0, -11.4) normal (0, 0, 1) x (1, 0, 0) in component "05 Rear electronics housing"
  line L0 (98.8, 33.8) -> (107.2, 33.8)
  line L1 (107.2, 33.8) -> (107.2, 42.2)
  line L2 (107.2, 42.2) -> (98.8, 42.2)
  line L3 (98.8, 42.2) -> (98.8, 33.8)
  dimension "d844" = 8.4
  dimension "d845" = 8.4
  measures "d844" horizontal distance of L0.start L0.end
  measures "d845" vertical distance of L0.end L1.end
extrude "Yoke mounting boss (1)" add sketch "Yoke mounting boss profile (1)" against normal blind 20.3 separate body makes body 100 in component "05 Rear electronics housing"
combine "Union manufactured solid (7)" operation add target body 66 tool bodies 100 in component "05 Rear electronics housing"
ref_plane "WorkPlane54" through (0, 0, -13.8) normal (0, 0, 1) x (1, 0, 0) in component "05 Rear electronics housing"
sketch "Yoke mounting boss hex pocket (1)" plane through (0, 0, -13.8) normal (0, 0, 1) x (1, 0, 0) in component "05 Rear electronics housing"
  line L0 (106.3486, 38) -> (104.6743, 40.9)
  line L1 (104.6743, 40.9) -> (101.3257, 40.9)
  line L2 (101.3257, 40.9) -> (99.6514, 38)
  line L3 (99.6514, 38) -> (101.3257, 35.1)
  line L4 (101.3257, 35.1) -> (104.6743, 35.1)
  line L5 (104.6743, 35.1) -> (106.3486, 38)
extrude "Yoke mounting boss hex pocket (2)" cut sketch "Yoke mounting boss hex pocket (1)" against normal blind 2.6 bodies 66 in component "05 Rear electronics housing"
ref_plane "WorkPlane55" through (0, 0, -13.8) normal (0, 0, 1) x (1, 0, 0) in component "05 Rear electronics housing"
sketch "Yoke mounting boss side nut entry profile (1)" plane through (0, 0, -13.8) normal (0, 0, 1) x (1, 0, 0) in component "05 Rear electronics housing"
  line L0 (98.5, 35.1) -> (103, 35.1)
  line L1 (103, 35.1) -> (103, 40.9)
  line L2 (103, 40.9) -> (98.5, 40.9)
  line L3 (98.5, 40.9) -> (98.5, 35.1)
  dimension "d854" = 4.5
  dimension "d855" = 5.8
  measures "d854" horizontal distance of L0.start L0.end
  measures "d855" vertical distance of L0.end L1.end
extrude "Yoke mounting boss side nut entry (1)" cut sketch "Yoke mounting boss side nut entry profile (1)" against normal blind 2.6 bodies 66 in component "05 Rear electronics housing"
ref_plane "WorkPlane56" through (0, 0, -11.38) normal (0, 0, 1) x (1, 0, 0) in component "05 Rear electronics housing"
sketch "Yoke mounting boss blind bore profile (1)" plane through (0, 0, -11.38) normal (0, 0, 1) x (1, 0, 0) in component "05 Rear electronics housing"
  circle A0 centre (103, 38) radius 1.7
  dimension "d860" = 3.4
  measures "d860" diameter of A0
extrude "Yoke mounting boss blind bore (1)" cut sketch "Yoke mounting boss blind bore profile (1)" against normal blind 6.82 bodies 66 in component "05 Rear electronics housing"
ref_plane "WorkPlane57" through (0, 0, -12.5) normal (0, 0, 1) x (1, 0, 0) in component "05 Rear electronics housing"